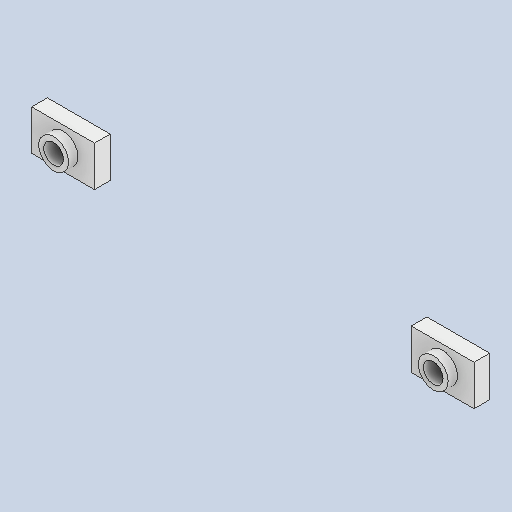
# Autodesk Inventor part: palito arriba de la banda
Saved by Autodesk Inventor 2025 (Build 290162000, 162)
## iProperties
Created: 2025-05-25
Part Number: palito arriba de la banda
Material: PVC, no plastificado
Document SubType Name: Modeling
Designer: STEVEN LONDOÑO
Density: 1.29 g/cm^3
Appearance: Suave - Blanco
Author: STEVEN LONDOÑO
Autodesk Inventor part; units mm, degrees
ref_plane "YZ Plane" through (0, 0, 0) normal (1, 0, 0) x (0, 1, 0)
ref_plane "XZ Plane" through (0, 0, 0) normal (0, 1, 0) x (-1, 0, 0)
ref_plane "XY Plane" through (0, 0, 0) normal (0, 0, 1) x (1, 0, 0)
sketch "Boceto1" plane through (0, 0, 0) normal (0, 0, 1) x (1, 0, 0)
  line L0 (-13.9318, 5.6251) -> (-13.9318, -7.1948)
  line L1 (-13.9318, -7.1948) -> (126.9482, -7.1948)
  line L2 (126.9482, -7.1948) -> (126.9482, 5.6251)
  line L3 (126.9482, 5.6251) -> (-13.9318, 5.6251)
  line L4 (126.9482, -7.1948) -> (116.9482, -7.1948)
  line L5 (116.9482, -7.1948) -> (116.9482, -0.7849)
  circle A0 centre (116.9482, -0.7849) radius 3.155
  line L6 (-13.9318, -7.1948) -> (-3.9318, -7.1948)
  line L7 (-3.9318, -7.1948) -> (-3.9318, -0.7849)
  circle A1 centre (-3.9318, -0.7849) radius 3.155
  circle A2 centre (-3.9318, -0.7849) radius 4.75
  circle A3 centre (116.9482, -0.7849) radius 4.75
  point P0 (0, 0)
  dimension "d1" = 10
  dimension "d2" = 6.31
  dimension "d4" = 6.31
  dimension "d5" = 6.41
  dimension "d6" = 6.41
  dimension "d7" = 9.5
  dimension "d8" = 9.5
  constraints: 16 end point, 4 centre point, 4 coincident, 3 perpendicular, 2 point on line, 2 vertical, 1 horizontal
  measures "d1" distance of L1.end L4.end
  measures "d2" diameter of A0
  measures "d4" diameter of A1
  measures "d5" distance from line of L3 A0.centre
  measures "d6" distance from line of L1 A1.centre
  measures "d7" diameter of A2
  measures "d8" diameter of A3
extrude "Extrusión1" add sketch "Boceto1" along normal blind 5 contours L3 L2 L1 L0
extrude "Extrusión2" add sketch "Boceto1" along normal blind 8 contours A2 | A3
sketch "Boceto2" plane through (-13.9318, -7.1948, 0) normal (0, -1, 0) x (1, 0, 0)
  line L0 (0, 0) -> (0, 5) projected
  line L1 (0, 0) -> (140.88, 0) projected
  line L2 (140.88, 0) -> (120.88, 0)
  line L3 (120.88, 0) -> (120.88, 5)
  line L4 (120.88, 5) -> (20, 5)
  line L5 (20, 5) -> (20, 0)
  point P0 (13.9318, 0)
  constraints: 8 end point, 2 perpendicular, 2 point on line, 1 parallel
extrude "Extrusión3" cut sketch "Boceto2" against normal through all
